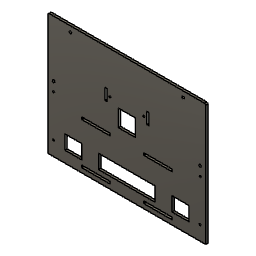
monitor_back_plate (Autodesk Fusion 360 design; units mm, degrees)
Autodesk Fusion 360 part; units mm, degrees
note: some values were not read from the file. Set by a fixed rule: the direction of a hole.
sketch "スケッチ1" plane through (0, 0, 0) normal (0, 0, 1) x (1, 0, 0)
  line L0 (140, 0) -> (140, 216)
  line L1 (140, 216) -> (-140, 216)
  line L2 (-140, 216) -> (-140, 0)
  line L3 (-39, 132) -> (-35, 132)
  line L4 (-35, 132) -> (-35, 152)
  line L5 (-35, 152) -> (-39, 152)
  line L6 (-39, 152) -> (-39, 132)
  line L7 (35, 132) -> (39, 132)
  line L8 (39, 132) -> (39, 152)
  line L9 (39, 152) -> (35, 152)
  line L10 (35, 152) -> (35, 132)
  line L11 (-140, 0) -> (140, 0)
  line L12 (-35, 142) -> (-30, 142)
  line L13 (35, 142) -> (30, 142)
  line L14 (-130, 116) -> (-130, 206)
  line L15 (-130, 206) -> (130, 206)
  line L16 (130, 206) -> (130, 116)
  line L17 (15, 132) -> (-15, 132)
  line L18 (-15, 132) -> (-15, 102)
  line L19 (-15, 102) -> (15, 102)
  line L20 (15, 102) -> (15, 132)
  line L21 (15, 132) -> (-15, 102) construction
  line L22 (-15, 132) -> (15, 102) construction
  line L23 (-140, 82) -> (140, 82)
  line L24 (-80, 82) -> (-30, 82)
  line L25 (-30, 82) -> (-30, 86)
  line L26 (-30, 86) -> (-80, 86)
  line L27 (-80, 86) -> (-80, 82)
  line L28 (30, 82) -> (80, 82)
  line L29 (80, 82) -> (80, 86)
  line L30 (80, 86) -> (30, 86)
  line L31 (30, 86) -> (30, 82)
  line L32 (-130, 0) -> (-130, 25.5)
  line L33 (130, 0) -> (130, 25.5)
  line L34 (-50, 20) -> (50, 20)
  line L35 (50, 20) -> (50, 45)
  line L36 (50, 45) -> (-50, 45)
  line L37 (-50, 45) -> (-50, 20)
  line L38 (80, 20) -> (110, 20)
  line L39 (110, 20) -> (110, 45)
  line L40 (110, 45) -> (80, 45)
  line L41 (80, 45) -> (80, 20)
  line L42 (-80, 8) -> (-30, 8)
  line L43 (-30, 8) -> (-30, 12)
  line L44 (-30, 12) -> (-80, 12)
  line L45 (-80, 12) -> (-80, 8)
  line L46 (30, 8) -> (80, 8)
  line L47 (80, 8) -> (80, 12)
  line L48 (80, 12) -> (30, 12)
  line L49 (30, 12) -> (30, 8)
  line L50 (-80, 20) -> (-110, 20)
  line L51 (-110, 20) -> (-110, 45)
  line L52 (-110, 45) -> (-80, 45)
  line L53 (-80, 45) -> (-80, 20)
  line L54 (-130, 82) -> (-130, 99.5)
  line L55 (130, 82) -> (130, 99.5)
  point P0 (0, 216)
  point P1 (-100, 206)
  point P2 (100, 206)
  point P3 (0, 117)
  point P4 (0, 20)
  dimension "d3" = 4
  dimension "d5" = 20
  dimension "d10" = 216
  dimension "d20" = 280
  dimension "d24" = 5
  dimension "d25" = 5
  dimension "d26" = 10
  dimension "d27" = 10
  dimension "d28" = 10
  dimension "d29" = 90
  dimension "d30" = 100
  dimension "d31" = 100
  dimension "d45" = 30
  dimension "d46" = 30
  dimension "d51" = 20
  dimension "d52" = 50
  dimension "d53" = 50
  dimension "d54" = 4
  dimension "d57" = 10
  dimension "d58" = 10
  dimension "d59" = 25.5
  dimension "d60" = 25.5
  dimension "d63" = 25
  dimension "d67" = 8
  dimension "d68" = 30
  dimension "d69" = 30
  dimension "d70" = 50
  dimension "d71" = 50
  dimension "d72" = 4
  dimension "d73" = 20
  dimension "d74" = 100
  dimension "d75" = 30
  dimension "d76" = 30
  dimension "d77" = 70
  dimension "d78" = 17.5
  dimension "d79" = 50
  dimension "d80" = 35
  dimension "d81" = 35
  dimension "d82" = 30
  dimension "d83" = 30
  constraint vertical L0
  constraint horizontal L1
  constraint vertical L2
  constraint horizontal L3
  constraint vertical L4
  constraint horizontal L5
  constraint vertical L6
  constraint horizontal L7
  constraint vertical L8
  constraint horizontal L9
  constraint vertical L10
  constraint collinear L5 L9
  constraint collinear L3 L7
  constraint equal L5 L9
  constraint midpoint L1 P0
  constraint perpendicular L2 L11
  constraint midpoint L4 L12.start
  constraint perpendicular L4 L12
  constraint midpoint L10 L13.start
  constraint perpendicular L10 L13
  constraint vertical L14
  constraint perpendicular L14 L15
  constraint perpendicular L15 L16
  constraint equal L14 L16
  constraint coincident L15 P1
  constraint coincident L15 P2
  constraint horizontal L17
  constraint perpendicular L17 L18
  constraint parallel L17 L19
  constraint parallel L18 L20
  constraint coincident L21 P3
  constraint coincident L22 P3
  constraint coincident L2 L23.start
  constraint coincident L0 L23.end
  constraint perpendicular L0 L23
  constraint horizontal L24
  constraint vertical L25
  constraint horizontal L26
  constraint vertical L27
  constraint coincident L23 L24.start
  constraint horizontal L28
  constraint vertical L29
  constraint horizontal L30
  constraint vertical L31
  constraint coincident L23 L28.start
  constraint collinear L26 L30
  constraint coincident L11 L32.start
  constraint perpendicular L11 L32
  constraint horizontal L34
  constraint vertical L35
  constraint horizontal L36
  constraint vertical L37
  constraint horizontal L38
  constraint vertical L39
  constraint horizontal L40
  constraint vertical L41
  constraint collinear L36 L40
  constraint collinear L34 L38
  constraint coincident origin L11
  constraint midpoint origin L11
  constraint coincident L0.start L11.end
  constraint horizontal L42
  constraint vertical L43
  constraint horizontal L44
  constraint vertical L45
  constraint horizontal L46
  constraint vertical L47
  constraint horizontal L48
  constraint vertical L49
  constraint horizontal L50
  constraint vertical L51
  constraint horizontal L52
  constraint vertical L53
  constraint collinear L36 L52
  constraint collinear L34 L50
  constraint midpoint L34 P4
  constraint vertical origin P4
  constraint collinear L44 L48
  constraint collinear L42 L46
  constraint coincident L23 L54.start
  constraint perpendicular L23 L54
  constraint coincident L23 L55.start
  constraint perpendicular L23 L55
  constraint collinear L32 L54
  constraint collinear L33 L55
  constraint equal L54 L55
  constraint vertical origin P3
  measures "d3" distance of L8.end L9.end
  measures "d5" distance of L7.end L8.end
  measures "d10" distance of origin L1
  measures "d20" distance of L0 L2
  measures "d24" distance of L12.start L12.end
  measures "d25" distance of L13.start L13.end
  measures "d26" distance of L1 L15
  measures "d27" distance of L2 L14
  measures "d28" distance of L0 L16
  measures "d29" distance of L14.start L14.end
  measures "d30" horizontal distance of P0 P2
  measures "d31" horizontal distance of P0 P1
  measures "d45" distance of L17.end L18.end
  measures "d46" distance of L17.start L17.end
  measures "d51" distance of L19 L23
  measures "d52" distance of L25.end L26.end
  measures "d53" distance of L29.end L30.end
  measures "d54" distance of L28.end L29.end
  measures "d57" distance of L2 L32
  measures "d58" distance of L0 L33
  measures "d59" distance of L32.start L32.end
  measures "d60" distance of L33.start L33.end
  measures "d63" distance of L38.start L40.end
  measures "d67" distance of L11 L42
  measures "d68" distance of origin L43
  measures "d69" distance of origin L49
  measures "d70" distance of L43.end L44.end
  measures "d71" distance of L47.end L48.end
  measures "d72" distance of L42.start L44.end
  measures "d73" distance of L11 L38
  measures "d74" distance of L35.end L36.end
  measures "d75" distance of L35 L41
  measures "d76" distance of L37 L53
  measures "d77" distance of L23 L44
  measures "d78" distance of L54.start L54.end
  measures "d79" distance of L7 L23
  measures "d80" distance of origin L10
  measures "d81" distance of origin L4
  measures "d82" distance of L51.end L52.end
  measures "d83" distance of L39.end L40.end
extrude "押し出し1" add sketch "スケッチ1" along normal blind 4 contours L0 L2 L11 L23 L24 L28 | L0 L1 L2 L23 L25 L26 L27 L29 L30 L31
hole "穴1" at (-30, 142, 0) at (30, 142, 0) at (-130, 25.5, 0) at (130, 25.5, 0) at (130, 99.5, 0) at (-130, 99.5, 0) direction (0, 0, 1) diameter 3.2 depth 35 tip angle 118
hole "穴2" at (-130, 116, 0) at (-100, 206, 0) at (100, 206, 0) at (130, 116, 0) direction (0, 0, 1) diameter 4.3 depth 35 tip angle 118
fillet "フィレット1" radius 2 2 edges at (140, 216, 2) (-140, 216, 2)
equation "d59 = 13.5 mm + 12 mm"
equation "d60 = 13.5 mm + 12 mm"
